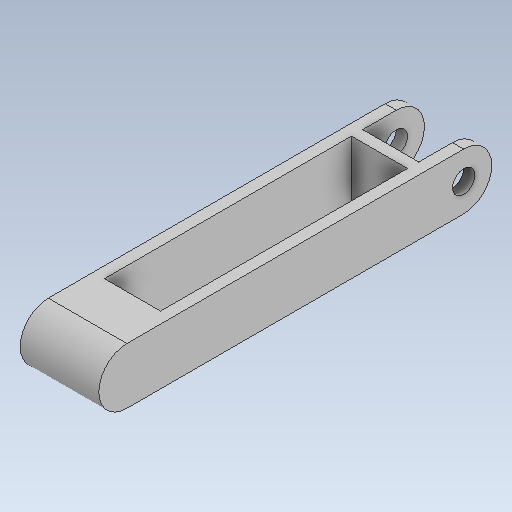
# Autodesk Inventor part: arm2
Saved by Autodesk Inventor 2020.3 (Build 243373000, 373)
## iProperties
Created: 2021-08-13
Part Number: arm2
Material: Generic
Document SubType Name: Modeling
Designer: 0x6f736f646f
Density: 1 g/cm^3
Appearance: Default
Mass: 507.074 g
Surface Area: 924.591 cm^2
Volume: 507.074 cm^3
Author: 0x6f736f646f
Autodesk Inventor part; units mm, degrees
ref_plane "YZ Plane" through (0, 0, 0) normal (1, 0, 0) x (0, 1, 0)
ref_plane "XZ Plane" through (0, 0, 0) normal (0, 1, 0) x (-1, 0, 0)
ref_plane "XY Plane" through (0, 0, 0) normal (0, 0, 1) x (1, 0, 0)
sketch "Sketch1" plane through (0, 0, 0) normal (1, 0, 0) x (0, 1, 0)
  line L0 (0, 0) -> (0, 300)
  circle A0 centre (0, 300) radius 25
  circle A1 centre (0, 0) radius 25
  circle A2 centre (0, 300) radius 10
  circle A3 centre (0, 0) radius 10
  line L1 (25, 300) -> (25, 0)
  line L2 (-25, 0) -> (-25, 300)
  dimension "d0" = 300
  dimension "d1" = 50
  dimension "d2" = 20
  constraints: 6 end point, 4 centre point, 4 coincident, 4 point on circle, 3 tangent, 2 equal radius, 1 parallel, 1 vertical
  measures "d0" distance of L0.start L0.end
  measures "d1" diameter of A0
  measures "d2" diameter of A2
extrude "Extrusion1" add sketch "Sketch1" along normal blind 70 contours A1 | A1 L2 A0 L0 | L0 A0 L1 A1 | A2 | A0
sketch "Sketch2" plane through (0, 25, 300) normal (0, 1, 0) x (1, 0, 0)
  line L0 (0, -25) -> (0, 0) projected
  line L1 (70, 300) -> (70, 325) projected
  line L2 (0, 0) -> (70, 0)
  line L3 (70, 0) -> (70, 300)
  line L4 (70, 300) -> (0, 300)
  line L5 (0, 300) -> (0, 0)
  line L6 (10, 10) -> (60, 10)
  line L7 (60, 10) -> (60, 290)
  line L8 (60, 290) -> (10, 290)
  line L9 (10, 290) -> (10, 10)
  line L10 (0, 325) -> (70, 325) projected
  line L11 (10, 290) -> (60, 290)
  line L12 (60, 290) -> (60, 325)
  line L13 (60, 325) -> (10, 325)
  line L14 (10, 325) -> (10, 290)
  line L15 (0, -25) -> (70, -25) projected
  line L16 (10, 10) -> (60, 10)
  line L17 (60, 10) -> (60, -25)
  line L18 (60, -25) -> (10, -25)
  line L19 (10, -25) -> (10, 10)
  line L20 (60, 260) -> (10, 260)
  line L21 (10, 260) -> (10, 40)
  line L22 (10, 40) -> (60, 40)
  line L23 (60, 40) -> (60, 260)
  line L24 (60, 325) -> (10, 325)
  line L25 (10, 325) -> (10, 270)
  line L26 (10, 270) -> (60, 270)
  line L27 (60, 270) -> (60, 325)
  line L28 (60, -25) -> (10, -25)
  line L29 (10, -25) -> (10, 30)
  line L30 (10, 30) -> (60, 30)
  line L31 (60, 30) -> (60, -25)
  point P0 (60, 40)
  point P1 (10, 260)
  point P2 (60, 270)
  dimension "d5" = 10
  dimension "d6" = 10
  dimension "d9" = 30
  dimension "d10" = 30
  dimension "d13" = 10
  dimension "d14" = 10
  constraints: 56 end point, 14 parallel, 7 perpendicular, 7 point on line, 6 horizontal, 3 other
  measures "d5" distance between parallel lines of L5 L9
  measures "d6" distance between parallel lines of L1 L17
  measures "d9" distance between parallel lines of L6 L22
  measures "d10" distance between parallel lines of L20 L8
  measures "d13" distance between parallel lines of L20 L26
  measures "d14" distance between parallel lines of L30 L22
extrude "Extrusion2" cut sketch "Sketch2" against normal through all contours L14 L10 L12 L4 | L4 L12 L8 L14 | L8 L7 L26 L9
extrude "Extrusion3" cut sketch "Sketch2" against normal through all contours L9 L20 L7 L22
body "Solid1"
